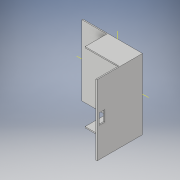
# Autodesk Inventor part: ProjectXBaseTop
Saved by Autodesk Inventor 2019.4 (Build 234330000, 330)
## iProperties
Created: 2021-04-19
Part Number: ProjectXBaseTop
Material: Generic
Document SubType Name: Modeling
Designer: ville
Density: 1 g/cm^3
Appearance: Default
Author: ville
Autodesk Inventor part; units mm, degrees
ref_plane "YZ Plane" through (0, 0, 0) normal (1, 0, 0) x (0, 1, 0)
ref_plane "XZ Plane" through (0, 0, 0) normal (0, 1, 0) x (-1, 0, 0)
sketch "Sketch2" plane through (0, 0, 0) normal (0, 0, 1) x (1, 0, 0)
  line L0 (-32.2657, 32.5) -> (21.7343, 32.5)
  line L1 (21.7343, 32.5) -> (21.7343, -32.5)
  line L2 (21.7343, -32.5) -> (-32.2657, -32.5)
  line L3 (-32.2657, -32.5) -> (-32.2657, 32.5)
  line L4 (-43.0657, 0) -> (32.5343, 0) projected
  point P0 (0, 0)
  dimension "d13" = 54
  dimension "d14" = 65
  constraints: 8 end point, 2 parallel, 1 horizontal, 1 perpendicular, 1 other
  measures "d13" distance of L1.end L2.end
  measures "d14" distance between parallel lines of L0 L2
extrude "Extrusion2" add sketch "Sketch2" along normal blind 1
sketch "Sketch3" plane through (21.7343, -32.5, 0) normal (1, 0, 0) x (0, 0, -1)
  line L0 (0, 0) -> (-21, 0)
  line L1 (-21, 0) -> (-21, 65)
  line L2 (-21, 65) -> (0, 65)
  line L3 (0, 65) -> (0, 0)
  line L4 (-1, 0) -> (-1, 65) projected
  line L5 (0, 65) -> (0, 0) projected
  line L6 (0, 65) -> (-1, 65) projected
  point P0 (0, 32.5)
  dimension "d9" = 20
  constraints: 8 end point, 2 collinear, 2 parallel, 1 horizontal, 1 perpendicular
  measures "d9" distance between parallel lines of L4 L1
extrude "Extrusion3" add sketch "Sketch3" along normal blind 1
sketch "Sketch4" plane through (21.7343, 32.5, 21) normal (0, 1, 0) x (1, 0, 0)
  line L0 (0, 20) -> (-54, 20) projected
  line L1 (0, 0) -> (0, 20) projected
  line L2 (-31, 20) -> (0, 20)
  line L3 (0, 20) -> (0, 0)
  line L4 (0, 0) -> (-31, 0)
  line L5 (-31, 0) -> (-31, 20)
  line L6 (1, 21) -> (1, 0) projected
  point P0 (-21.7343, 21)
  dimension "d15" = 32
  constraints: 8 end point, 2 parallel, 1 horizontal, 1 perpendicular, 1 point on line
  measures "d15" distance between parallel lines of L6 L5
extrude "Extrusion4" add sketch "Sketch4" against normal blind 1
ref_plane "Work Plane2" through (21.7343, 0, 1) normal (0, -1, 0) x (1, 0, 0)
mirror "Mirror3" about plane through (21.7343, 0, 1) normal (0, -1, 0) of "Extrusion4"
sketch "Sketch5" plane through (22.7343, -32.5, 21) normal (0, 0, 1) x (1, 0, 0)
  line L0 (-1, 64) -> (-32, 64) projected
  line L1 (-1, 64) -> (-1, 65)
  line L2 (-55, 65) -> (0, 65) projected
  line L3 (-32, 1) -> (-1, 1) projected
  line L4 (-1, 1) -> (-1, 0)
  line L5 (0, 0) -> (-55, 0) projected
  line L6 (-1, 1) -> (-1, 64) projected
  line L7 (0, 65) -> (0, 0) projected
  line L8 (0, 65) -> (-32, 65) projected
  line L9 (0, 0) -> (-32, 0) projected
  point P0 (-22.7343, 32.5)
  constraints: 4 end point, 3 point on line, 1 vertical
extrude "Extrusion5" add sketch "Sketch5" along normal blind 21
sketch "Sketch6" plane through (22.7343, -32.5, 0) normal (1, 0, 0) x (0, 0, -1)
  line L0 (-35, 37.5) -> (-40, 37.5)
  line L1 (-40, 37.5) -> (-40, 27.5)
  line L2 (-40, 27.5) -> (-35, 27.5)
  line L3 (-35, 27.5) -> (-35, 37.5)
  line L4 (-42, 0) -> (-42, 65) projected
  line L5 (0, 32.5) -> (-42, 32.5) construction
  dimension "d18" = 2
  dimension "d19" = 5
  dimension "d20" = 10
  constraints: 10 end point, 2 parallel, 1 horizontal, 1 midpoint, 1 perpendicular, 1 other
  measures "d18" distance between parallel lines of L1 L4
  measures "d19" distance of L0.start L0.end
  measures "d20" distance between parallel lines of L2 L0
extrude "Extrusion6" cut sketch "Sketch6" against normal up to next
body "Solid2"
